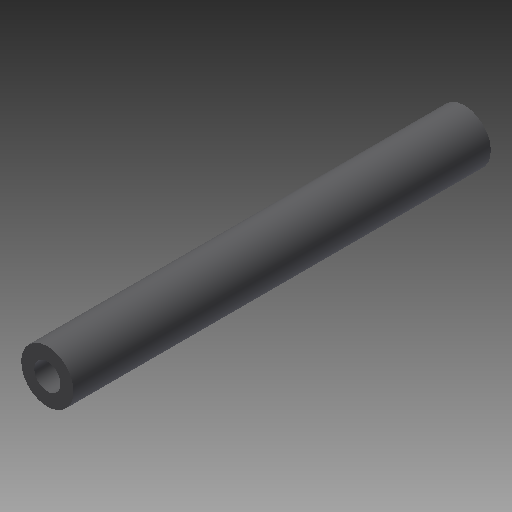
# Autodesk Inventor part: POST0.75-1.872
Saved by Autodesk Inventor 2017 (Build 210142000, 142)
## iProperties
Category: PARTsolutions
Company: BIMBA
Created: 2017-01-25
Part Number: POST0.75-1.872
Catalog Web Link: www.cadenas.de
Description: BIF Post-Bimba FLAT-1
Vendor: BIMBA
Document SubType Name: Modeling
Designer: psAdmin
Manufacturer: BIMBA
Mass: 0.995079 g
Surface Area: 13.8122 cm^2
Volume: 0.995079 cm^3
Density: 1 g/cm^3
Material: Generic
Appearance: PSOLRGB-192-192-192
PSOL_IDENT_0: {$CADENAS_DATA\23d-libs\bimba\bimba\bimba_imperial\bimba_full_line\flat_cylinders\fo1\bif_post.prj},
PSOL_IDENT_1: 176 {VTYP=3D},{NB=POST0.75-1.872},{LINA=POST0.75-1.872},{NN=BIF Post},{DATE=01.12.2016 06:16:11},{GE
PSOL_IDENT_2: OMDATE=24.05.2016 08:21:00},{VERSION=},{LINEID=90},{LINESUBID=-1},{WBVAR=L,AB}  {NB=POST0.75-1.872},
PSOL_IDENT_3: {LINA=POST0.75-1.872},{KT=DUMMY},{PN=POST0.75-1.872},{BORE=0.7500},{L=1.87200},{AB=},{DIA=0.235},{ID=
PSOL_IDENT_4: 0.11800}
NN: BIF Post
NT: Bimba FLAT-1
NB: POST0.75-1.872
NBSYN: $PN.
LINA: POST0.75-1.872
PN: POST0.75-1.872
BORE: 0.7500
L: 1.87200
AB: Standard
SUPPLIER: BIMBA
ARTICLENO: POST0.75-1.872
BOMINFO: POST0.75-1.872
CREATOR: CADENAS GmbH
Title: POST0.75-1.872
Author: Cadenas PARTsolutions
Comments: Bimba FLAT-1
Autodesk Inventor part; units mm, degrees
sketch "Sketch_1" plane through (0, 0, 0) normal (1, 0, 0) x (0, 1, 0)
  line L0 (0, -47.5488) -> (0, 0)
  line L1 (0, 0) -> (2.9845, 0)
  line L2 (2.9845, 0) -> (2.9845, -47.5488)
  line L3 (2.9845, -47.5488) -> (0, -47.5488)
  line L4 (0, -47.5488) -> (0, 0)
  constraints: 10 end point
revolve "Revolution1" add sketch "Sketch_1" angle 360 about axis through (0, 0, -47.5488) along (0, 0, -1)
sketch "Sketch2" plane through (0, 0, 0) normal (0, 0, 1) x (1, 0, 0)
  point P0 (0, 0)
hole "Hole1" at (0, 0, 0) direction (0, 0, -1) diameter 2.9972 depth 47.5488
ref_plane "screw_XY" through (0, 0, 0) normal (0, 0, 1) x (1, 0, 0)
ref_plane "screw_YZ" through (0, 0, 0) normal (1, 0, 0) x (0, 1, 0)
ref_plane "screw_ZX" through (0, 0, 0) normal (0, 1, 0) x (0, 0, 1)
body "Solid1"
